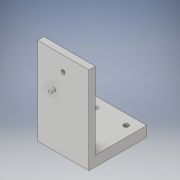
# Autodesk Inventor part: Middle Gear Frame
Saved by Autodesk Inventor 2017 (Build 210142000, 142)
## iProperties
Created: 2018-03-09
Part Number: Middle Gear Frame
Material: Generic
Document SubType Name: Modeling
Designer: Russ
Density: 1 g/cm^3
Appearance: Default
Author: Russ
Autodesk Inventor part; units mm, degrees
ref_plane "YZ Plane" through (0, 0, 0) normal (1, 0, 0) x (0, 1, 0)
ref_plane "XZ Plane" through (0, 0, 0) normal (0, 1, 0) x (-1, 0, 0)
ref_plane "XY Plane" through (0, 0, 0) normal (0, 0, 1) x (1, 0, 0)
sketch "Sketch1" plane through (0, 0, 0) normal (0, 0, 1) x (1, 0, 0)
  circle A0 centre (1.016, 27.4993) radius 1.905
  arc A1 (-3.2174, 19.2546) -> (-0.4706, 18.1168) centre (1.016, 25.5904) ccw
  circle A2 centre (1.016, 25.5904) radius 7.62
  arc A3 (-0.4706, -2.0514) -> (-3.2174, -3.1892) centre (1.016, -9.525) ccw
  arc A4 (2.5026, -16.9986) -> (5.2494, -15.8608) centre (1.016, -9.525) ccw
  circle A5 centre (1.016, -9.525) radius 7.62
  line L0 (1.016, -1.905) -> (1.016, 17.9704)
  circle A6 centre (1.016, 8.0327) radius 9.525
  line L1 (0, 16.0654) -> (2.032, 16.0654)
  line L2 (2.032, 0) -> (0, 0)
  circle A7 centre (-7.874, 8.0327) radius 9.525
  line L3 (26.416, 41.9773) -> (-24.384, 41.9773)
  line L4 (-24.384, -44.2811) -> (-24.384, 41.9773)
  line L5 (26.416, -44.2811) -> (26.416, 41.9773)
  line L6 (-75.184, -44.2811) -> (77.216, -44.2811)
  line L7 (1.016, 8.0327) -> (-47.2731, 8.0327)
  circle A8 centre (-24.384, 8.0327) radius 21.5247
  circle A9 centre (1.016, -9.525) radius 1.905
  circle A10 centre (-7.874, 8.0327) radius 1.905
  point P0 (0, 0)
  dimension "d0" = 19.05
  dimension "d1" = 19.05
  dimension "d2" = 8.89
  dimension "d3" = 3.81
  dimension "d4" = 3.81
  dimension "d5" = 3.81
  dimension "d32" = 71.7804
  dimension "d33" = 44.2811
  dimension "d34" = 25.4
  dimension "d35" = 0
  dimension "d36" = 0
  dimension "d37" = 86.2584
  constraints: 16 end point, 9 centre point, 6 point on circle, 5 coincident, 2 point on line, 2 vertical alignment, 1 horizontal, 1 midpoint, 1 vertical, 4 other
  measures "d0" diameter of A6
  measures "d1" diameter of A7
  measures "d2" distance from line of L0 A7.centre
  measures "d3" diameter of A9
  measures "d4" diameter of A0
  measures "d5" diameter of A10
  measures "d32" distance from line of L6 A0.centre
  measures "d33" distance from line of L6 point (0, 0)
  measures "d34" distance from line of L4 A0.centre
  measures "d35" distance from line of L6 L5.start
  measures "d36" distance from line of L6 L4.start
  measures "d37" distance between parallel lines of L3 L6
extrude "Extrusion1" add sketch "Sketch1" along normal blind 6.35 contours A2 A1 | A5 A4 A3 | A6 A7 A8 L4 L3 L5 L6 | A7 A8 A6 | A6 A8 L7 L0 A7 | L0 A7 | A8 A7 L7 A10 A6 | A6 A10 L7 A8 | A8 L4 L7 A7 | L7 A8 A6 A7 L0 | L7 A10 A6 A8 | L7 L4 A8 A7 | A7 A8 A6 A10 L7 | A6 A8 A7 | A9
sketch "Sketch2" plane through (0, 0, 6.35) normal (0, 0, 1) x (1, 0, 0)
  line L0 (-3.429, -3.0002) -> (13.2364, -3.0002)
  line L1 (13.2364, -3.0002) -> (13.2364, 18.7074)
  line L2 (13.2364, 18.7074) -> (-3.429, 18.7074)
  line L3 (-3.429, 18.7074) -> (-3.429, -3.0002)
  point P0 (0, 0)
  constraints: 8 end point, 2 parallel, 1 horizontal, 1 perpendicular
extrude "Extrusion2" add sketch "Sketch2" against normal blind 6.35
sketch "Sketch3" plane through (0, 0, 0) normal (0, 0, -1) x (-1, 0, 0)
  line L0 (24.384, 41.9773) -> (24.384, -44.2811) projected
  line L1 (-26.416, -44.2811) -> (24.384, -44.2811)
  line L2 (24.384, -44.2811) -> (24.384, -34.1211)
  line L3 (24.384, -34.1211) -> (-26.416, -34.1211)
  line L4 (-26.416, -34.1211) -> (-26.416, -44.2811)
  point P0 (0, 0)
  dimension "d10" = 10.16
  constraints: 8 end point, 2 parallel, 1 horizontal, 1 perpendicular, 1 point on line
  measures "d10" distance between parallel lines of L1 L3
extrude "Extrusion3" add sketch "Sketch3" along normal blind 50.8
sketch "Sketch4" plane through (-24.384, -34.1211, 0) normal (0, 1, 0) x (1, 0, 0)
  circle A0 centre (40.64, 40.64) radius 2.3813
  circle A1 centre (10.16, 40.64) radius 2.3813
  line L0 (50.8, 0) -> (0, 0)
  line L1 (0, 50.8) -> (50.8, 50.8) projected
  line L2 (50.8, 0) -> (50.8, 50.8) projected
  line L3 (0, 0) -> (0, 50.8) projected
  point P0 (24.384, 0)
  dimension "d13" = 4.7625
  dimension "d14" = 4.7625
  dimension "d17" = 10.16
  dimension "d18" = 10.16
  dimension "d19" = 10.16
  dimension "d20" = 10.16
  constraints: 2 centre point, 2 end point
  measures "d13" diameter of A1
  measures "d14" diameter of A0
  measures "d17" distance from line of L1 A0.centre
  measures "d18" distance from line of L2 A0.centre
  measures "d19" distance from line of L1 A1.centre
  measures "d20" distance from line of L3 A1.centre
extrude "Extrusion4" cut sketch "Sketch4" against normal up to next contours A0 | A1
sketch "Sketch5" plane through (0, 0, 6.35) normal (0, 0, 1) x (1, 0, 0)
  circle A0 centre (-7.874, 8.0327) radius 1.905 projected
  point P0 (0, 0)
extrude "Extrusion5" add sketch "Sketch5" against normal blind 6.35
sketch "Sketch6" plane through (0, 0, 6.35) normal (0, 0, 1) x (1, 0, 0)
  circle A0 centre (-7.874, 8.0327) radius 1.6256
  point P0 (0, 0)
  dimension "d27" = 3.2512
  dimension "d28" = 8.0327
  dimension "d29" = 7.874
  constraints: 1 centre point
  measures "d27" diameter of A0
  measures "d28" vertical distance of point (0, 0) A0.centre
  measures "d29" horizontal distance of point (0, 0) A0.centre
extrude "Extrusion6" add sketch "Sketch6" along normal blind 4.191
body "Solid1"
